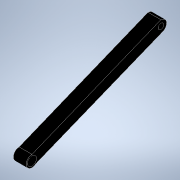
# Autodesk Inventor part: SLIDER CRANK LONG BAR
Saved by Autodesk Inventor 2021 (Build 250183000, 183)
## iProperties
Created: 2021-07-25
Part Number: SLIDER CRANK LONG BAR
Material: Generic
Document SubType Name: Modeling
Designer: HP
Density: 1 g/cm^3
Appearance: Anodized - Black
Author: HP
Autodesk Inventor part; units mm, degrees
ref_plane "YZ Plane" through (0, 0, 0) normal (1, 0, 0) x (0, 1, 0)
ref_plane "XZ Plane" through (0, 0, 0) normal (0, 1, 0) x (-1, 0, 0)
ref_plane "XY Plane" through (0, 0, 0) normal (0, 0, 1) x (1, 0, 0)
sketch "Sketch1" plane through (0, 0, 0) normal (1, 0, 0) x (0, 1, 0)
  circle A0 centre (-9.525, 25.4) radius 1.5875
  circle A1 centre (-9.525, 25.4) radius 1.2319
  circle A2 centre (4.7625, -9.9196) radius 0.762
  circle A3 centre (4.7625, -9.9196) radius 1.5875
  line L0 (6.35, -9.9196) -> (-7.9375, 25.4)
  line L1 (-11.1125, 25.4) -> (3.2891, -10.5105)
  point P0 (0, 0)
  point P1 (-10.6726, 24.3031)
  dimension "d0" = 3.175
  dimension "d1" = 2.4638
  dimension "d11" = 1.524
  dimension "d12" = 3.175
  constraints: 4 centre point, 4 end point, 4 point on circle, 2 coincident, 1 tangent
  measures "d0" diameter of A0
  measures "d1" diameter of A1
  measures "d11" diameter of A2
  measures "d12" diameter of A3
extrude "Extrusion1" add sketch "Sketch1" along normal blind 3.5306 contours A0 L1 | L0 A3 L1 A0 | L1 A0 | L0 A3 picked at (5.8969, -9.4336)
body "Solid1"
